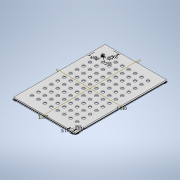
# Autodesk Inventor part: DSC pan lid carrier
Saved by Autodesk Inventor 2020 (Build 240168000, 168)
## iProperties
Created: 2021-10-05
Part Number: DSC pan lid carrier
Material: Generic
Document SubType Name: Modeling
Designer: pab2
Density: 1 g/cm^3
Appearance: Default
Author: pab2
Autodesk Inventor part; units mm, degrees
ref_plane "YZ Plane" through (0, 0, 0) normal (1, 0, 0) x (0, 1, 0)
ref_plane "XZ Plane" through (0, 0, 0) normal (0, 1, 0) x (-1, 0, 0)
ref_plane "XY Plane" through (0, 0, 0) normal (0, 0, 1) x (1, 0, 0)
sketch "Sketch1" plane through (0, 0, 0) normal (0, 1, 0) x (-1, 0, 0)
  line L0 (0, 0) -> (-85.471, 0)
  line L1 (-85.471, 0) -> (-85.471, 127.762)
  line L2 (-85.471, 127.762) -> (0, 127.762)
  line L3 (0, 127.762) -> (0, 0)
  line L4 (-85.471, 127.762) -> (-80.7085, 127.762)
  line L5 (-80.7085, 127.762) -> (-80.7085, 122.9995)
  line L6 (-80.7085, 122.9995) -> (-85.471, 122.9995)
  line L7 (-85.471, 122.9995) -> (-85.471, 127.762)
  line L8 (0, 0) -> (-11.2522, 0)
  line L9 (-11.2522, 0) -> (-11.2522, 14.3764)
  line L10 (-11.2522, 14.3764) -> (0, 14.3764)
  line L11 (0, 14.3764) -> (0, 0)
  circle A0 centre (-11.2522, 14.3764) radius 3.75
  circle A1 centre (-11.2522, 14.3764) radius 2
  circle A2 centre (-80.7085, 122.9995) radius 1.25
  point P0 (-42.7355, 0)
  point P1 (0, 63.881)
  dimension "d0" = 85.471
  dimension "d1" = 127.762
  dimension "d20" = 4.7625
  dimension "d21" = 4.7625
  dimension "d29" = 11.2522
  dimension "d30" = 14.3764
  dimension "d31" = 7.5
  dimension "d32" = 4
  dimension "d35" = 2.5
  constraints: 24 end point, 6 parallel, 3 centre point, 3 coincident, 3 horizontal, 3 perpendicular, 2 midpoint
  measures "d0" distance of L1.end L2.end
  measures "d1" distance of L0.end L1.end
  measures "d20" distance of L5.end L6.end
  measures "d21" distance of L4.end L5.end
  measures "d29" distance of L9.end L10.end
  measures "d30" distance of L8.end L9.end
  measures "d31" diameter of A0
  measures "d32" diameter of A1
  measures "d35" diameter of A2
extrude "Extrusion1" add sketch "Sketch1" along normal blind 2
sketch "Sketch2" plane through (0, 2, 0) normal (0, 1, 0) x (1, 0, 0)
  line L0 (85.471, 0) -> (0, 0) projected
  line L1 (0, 0) -> (11.2395, 0)
  line L2 (11.2395, 0) -> (11.2395, -14.3789)
  line L3 (11.2395, -14.3789) -> (0, -14.3789)
  line L4 (0, -14.3789) -> (0, 0)
  circle A0 centre (11.2395, -14.3789) radius 3.5
  dimension "d4" = 11.2395
  dimension "d5" = 14.3789
  dimension "d6" = 7
  constraints: 8 end point, 2 parallel, 1 centre point, 1 coincident, 1 horizontal, 1 perpendicular
  measures "d4" distance of L2.end L3.end
  measures "d5" distance of L1.end L2.end
  measures "d6" diameter of A0
hole "Hole1" at (11.2395, 2, 14.3789) direction (0, -1, 0) diameter 4 end through all
extrude "Extrusion2" cut sketch "Sketch1" along normal blind 1 contours A0 L10 A1 L9 | L9 A1 L10 A0 | A1 L10 L9 | L9 L10 A1
pattern_linear "Rectangular Pattern1" count 8 spacing 9 along (1, 0, 0) count 12 spacing 9 along (0, 0, 1) of "Hole1", "Extrusion2"
ref_plane "Work Plane1" through (42.7355, 0, 0) normal (1, 0, 0) x (0, 0, -1)
ref_plane "Work Plane2" through (0, 0, 63.881) normal (0, 0, -1) x (-1, 0, 0)
extrude "Extrusion3" add sketch "Sketch1" against normal blind 2 contours A2 L5 L6 | L6 L5 A2
mirror "Mirror1" about plane through (0, 0, 63.881) normal (0, 0, -1) of "Extrusion3"
mirror "Mirror2" about plane through (42.7355, 0, 0) normal (1, 0, 0) of "Mirror1", "Extrusion3"
body "Solid1"
